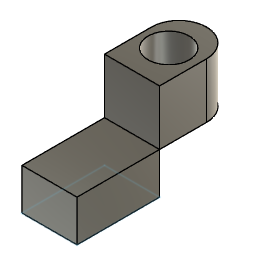
tamper for brick mold (Autodesk Fusion 360 design; units mm, degrees)
part number: 2025-07-14-21-31-38-461
part number: 2025-07-14-21-33-05-556
Autodesk Fusion 360 part; units mm, degrees
sketch "Sketch1" plane through (0, 0, 0) normal (0, 0, 1) x (1, 0, 0) in component "Tamper"
  line L0 (75.3462, 85.8858) -> (115.3462, 85.8858)
  line L1 (115.3462, 85.8858) -> (115.3462, 25.8858)
  line L2 (115.3462, 25.8858) -> (75.3462, 25.8858)
  line L3 (75.3462, 25.8858) -> (75.3462, 85.8858)
  dimension "d1" = 60
  dimension "d2" = 40
  constraint horizontal L0
  constraint vertical L1
  constraint horizontal L2
  constraint vertical L3
  measures "d1" distance of L0.start L2.end
  measures "d2" distance of L0.start L0.end
extrude "Extrude1" add sketch "Sketch1" along normal blind 30 makes body 1 in component "Tamper"
sketch "Sketch2" plane through (0, 0, 30) normal (0, 0, 1) x (-1, 0, 0) in component "Tamper"
  line L0 (-75.3462, -25.8858) -> (-115.3462, -25.8858)
  line L1 (-115.3462, -25.8858) -> (-115.3462, -85.8858)
  line L2 (-115.3462, -85.8858) -> (-75.3462, -85.8858)
  line L3 (-75.3462, -85.8858) -> (-75.3462, -25.8858)
  line L4 (-75.3462, -85.8858) -> (-75.3462, -120)
  line L5 (-115.3462, -85.8858) -> (-115.3462, -120)
  arc A0 (-115.3462, -120) -> (-75.3462, -120) centre (-95.3462, -120) ccw
  constraint coincident L2.end L3.start
  constraint perpendicular L2 L4
  constraint coincident L1.end L2.start
  constraint perpendicular L2 L5
  constraint tangent L4 A0
  constraint tangent L5 A0
extrude "Extrude2" add sketch "Sketch2" along normal blind 20 contours L2 L4 L5 A0 bodies 1 in component "Tamper"
hole "Hole1" at (94.7606, 113.1123, 50) direction (0, 0, -1) diameter 30 depth 20 tip angle 118 bodies 1 in component "Tamper"
extrude "Extrude3" add sketch "Sketch1" along normal blind 30 separate body makes body 2 in component "Tamper"
extrude "Extrude4" add 1 faces at (95.151, 89.9613, 50) along direction (0, 0, 1) blind 20 on bodies 1 bodies 1 in component "Tamper"
component "Tamper" placed x (1, 0, 0) y (0, 1, 0) z (0, 0, 1) at (0, 0, 0)
